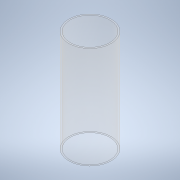
# Autodesk Inventor part: HSI
Saved by Autodesk Inventor 2022 (Build 260153000, 153)
## iProperties
Created: 2022-03-30
Part Number: HSI
Material: Polycarbonate, Clear
Document SubType Name: Modeling
Designer: RNG3nius
Density: 1.2 g/cm^3
Appearance: Polycarbonate - Clear
Mass: 74.1116 g
Surface Area: 571.047 cm^2
Volume: 61.7597 cm^3
Author: RNG3nius
Autodesk Inventor part; units mm, degrees
ref_plane "YZ Plane" through (0, 0, 0) normal (1, 0, 0) x (0, 1, 0)
ref_plane "XZ Plane" through (0, 0, 0) normal (0, 1, 0) x (-1, 0, 0)
ref_plane "XY Plane" through (0, 0, 0) normal (0, 0, 1) x (1, 0, 0)
sketch "Sketch5" plane through (0, 0, 0) normal (0, 1, 0) x (-1, 0, 0)
  circle A0 centre (0, 0) radius 28.8
  circle A1 centre (0, 0) radius 26.8
  dimension "d26" = 57.6
  dimension "d27" = 53.6
  constraints: 2 centre point, 2 coincident
  measures "d26" diameter of A0
  measures "d27" diameter of A1
extrude "Extrusion3" add sketch "Sketch5" along normal blind 138.4
body "Solid2"
